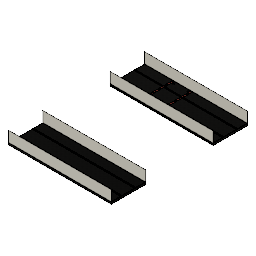
_6-9 (Long Straight 2).344d3e92-f278-4324-a628-1e91485c0ac5 (Autodesk Fusion 360 design; units mm, degrees)
Autodesk Fusion 360 part; units mm, degrees
note: some values were not read from the file. Chosen so that the rebuilt part matches the saved one: which bodies a step acts on.
sketch "Sketch1" plane through (0, 0, 0) normal (0, 0, 1) x (1, 0, 0)
  line L0 (0, 0) -> (0, -812.8)
  line L1 (0, -812.8) -> (0, -2413)
  line L2 (0, -2413) -> (0, -3225.8)
  line L3 (0, 0) -> (1219.2, 0)
  line L4 (1219.2, 0) -> (0, 0)
  line L5 (0, 0) -> (0, -812.8)
  line L6 (0, -812.8) -> (1219.2, -812.8)
  line L7 (1219.2, -812.8) -> (1219.2, 0)
  line L8 (0, -3225.8) -> (1219.2, -3225.8)
  line L9 (1219.2, -3225.8) -> (0, -3225.8)
  line L10 (0, -3225.8) -> (0, -2413)
  line L11 (0, -2413) -> (1219.2, -2413)
  line L12 (1219.2, -2413) -> (1219.2, -3225.8)
  dimension "d1" = 812.8
  dimension "d2" = 1600.2
  dimension "d3" = 812.8
  dimension "d4" = 1219.2
  dimension "d5" = 1219.2
  constraint coincident L0.start L3.start
  constraint vertical L0
  constraint parallel L0 L1
  constraint parallel L1 L2
  constraint perpendicular L0 L3
  constraint horizontal L4
  constraint vertical L5
  constraint horizontal L6
  constraint vertical L7
  constraint perpendicular L2 L8
  constraint horizontal L9
  constraint vertical L10
  constraint horizontal L11
  constraint vertical L12
  measures "d1" distance of L0.start L0.end
  measures "d2" distance of L0.end L1.end
  measures "d3" distance of L1.end L2.end
  measures "d4" distance of L0.start L3.end
  measures "d5" distance of L2.end L8.end
extrude "Extrude1" add sketch "Sketch1" along normal blind 50.8 makes body 1 at (406.4, -270.9333, 0) makes body 2 at (812.8, -2954.8667, 0)
sketch "Sketch2" plane through (0, 0, 50.8) normal (0, 0, 1) x (-1, 0, 0)
  line L0 (-1219.2, 2413) -> (0, 2413)
  line L1 (0, 2413) -> (0, 3225.8)
  line L2 (0, 3225.8) -> (-1219.2, 3225.8)
  line L3 (-1219.2, 3225.8) -> (-1219.2, 2413)
  line L4 (-106.2446, 261.963) -> (-283.0518, 261.963) construction
  line L5 (-283.0518, 261.963) -> (-283.0518, 108.5567) construction
  line L6 (-283.0518, 108.5567) -> (-106.2446, 108.5567) construction
  line L7 (-106.2446, 108.5567) -> (-106.2446, 261.963) construction
  dimension "d8" = 152.4
sketch "Sketch3" plane through (0, 0, 50.8) normal (0, 0, 1) x (-1, 0, 0)
  line L0 (-1219.2, 812.8) -> (-1219.2, 0)
  line L1 (-1219.2, 0) -> (0, 0)
  line L2 (0, 0) -> (0, 812.8)
  line L3 (0, 812.8) -> (-1219.2, 812.8)
  line L4 (-1219.2, 406.4) -> (-1139.825, 406.4)
  line L5 (-1139.825, 406.4) -> (-1111.25, 406.4)
  line L6 (-1111.25, 406.4) -> (-1111.25, 0)
  line L7 (-1111.25, 0) -> (-1139.825, 0)
  line L8 (-1139.825, 0) -> (-1139.825, 406.4)
  line L9 (-1139.825, 406.4) -> (-1111.25, 406.4)
  line L10 (-1111.25, 406.4) -> (-1111.25, 812.8)
  line L11 (-1111.25, 812.8) -> (-1139.825, 812.8)
  line L12 (-1139.825, 812.8) -> (-1139.825, 406.4)
  line L13 (-1219.2, 406.4) -> (-704.85, 406.4)
  line L14 (-704.85, 406.4) -> (-676.275, 406.4)
  line L15 (-676.275, 406.4) -> (-676.275, 0)
  line L16 (-676.275, 0) -> (-704.85, 0)
  line L17 (-704.85, 0) -> (-704.85, 406.4)
  line L18 (-676.275, 406.4) -> (-704.85, 406.4)
  line L19 (-704.85, 406.4) -> (-704.85, 812.8)
  line L20 (-704.85, 812.8) -> (-676.275, 812.8)
  line L21 (-676.275, 812.8) -> (-676.275, 406.4)
  dimension "d9" = 79.375
  dimension "d10" = 28.575
  dimension "d11" = 28.575
  dimension "d12" = 514.35
  dimension "d13" = 28.575
  dimension "d14" = 28.575
  constraint midpoint L0 L4.start
  constraint perpendicular L0 L4
  constraint horizontal L5
  constraint vertical L6
  constraint horizontal L7
  constraint vertical L8
  constraint coincident L1 L6.end
  constraint horizontal L9
  constraint vertical L10
  constraint horizontal L11
  constraint vertical L12
  constraint coincident L3 L10.end
  constraint perpendicular L12 L13
  constraint horizontal L14
  constraint vertical L15
  constraint horizontal L16
  constraint vertical L17
  constraint horizontal L18
  constraint vertical L19
  constraint horizontal L20
  constraint vertical L21
  measures "d9" distance of L4.start L4.end
  measures "d10" distance of L4.end L5.end
  measures "d11" distance of L4.end L5.end
  measures "d12" distance of L4.start L13.end
  measures "d13" distance of L13.end L14.end
  measures "d14" distance of L14.end L13.end
extrude "Extrude2" add sketch "Sketch3" along normal blind 0.0254 contours L3 L5 L9 L10 L11 L12 L13 | L1 L5 L6 L7 L8 L9 L13 | L3 L14 L18 L19 L20 L21 | L1 L14 L15 L16 L17 L18 bodies 1
sketch "Sketch4" plane through (0, 0, 50.8) normal (0, 0, 1) x (-1, 0, 0)
  line L0 (-676.275, 812.8) -> (-676.275, 0)
  line L1 (-676.275, 0) -> (0, 0)
  line L2 (0, 0) -> (0, 812.8)
  line L3 (0, 812.8) -> (-676.275, 812.8)
  line L4 (-1111.25, 812.8) -> (-1111.25, 0)
  line L5 (-1111.25, 0) -> (-704.85, 0)
  line L6 (-704.85, 0) -> (-704.85, 812.8)
  line L7 (-704.85, 812.8) -> (-1111.25, 812.8)
  line L8 (-1139.825, 0) -> (-1139.825, 812.8)
  line L9 (-1139.825, 812.8) -> (-1219.2, 812.8)
  line L10 (-1219.2, 812.8) -> (-1219.2, 0)
  line L11 (-1219.2, 0) -> (-1139.825, 0)
  line L12 (-704.85, 0) -> (-1111.25, 0)
  line L13 (-1111.25, 0) -> (-1111.25, 57.15)
  line L14 (-704.85, 57.15) -> (-704.85, 0)
  line L15 (-704.85, 812.8) -> (-1111.25, 812.8)
  line L16 (-1111.25, 812.8) -> (-1111.25, 755.65)
  line L17 (-704.85, 755.65) -> (-704.85, 812.8)
  circle A0 centre (-742.95, 57.15) radius 16
  circle A1 centre (-1085.85, 57.15) radius 16
  circle A2 centre (-742.95, 755.65) radius 16
  circle A3 centre (-1085.85, 755.65) radius 16
  dimension "d19" = 57.15
  dimension "d20" = 57.15
  dimension "d21" = 32
  dimension "d22" = 32
  dimension "d23" = 32
  dimension "d24" = 32
  constraint horizontal L12
  constraint vertical L13
  constraint vertical L14
  constraint coincident L5.end L6.start
  constraint horizontal L15
  constraint vertical L16
  constraint vertical L17
  constraint coincident L6.end L7.start
  measures "d19" distance of L5.end L14.start
  measures "d20" distance of L6.end L17.start
  measures "d21" diameter of A0
  measures "d22" diameter of A1
  measures "d23" diameter of A2
  measures "d24" diameter of A3
extrude "Extrude3" add sketch "Sketch4" along normal blind 0.0254 contours A0 | A1 | A2 | A3 bodies 1
sketch "Sketch5" plane through (0, 0, 50.8) normal (0, 0, 1) x (-1, 0, 0)
sketch "Sketch6" plane through (0, 0, 50.8) normal (0, 0, 1) x (-1, 0, 0)
  line L0 (-676.275, 812.8) -> (-676.275, 0)
  line L1 (-676.275, 0) -> (0, 0)
  line L2 (0, 0) -> (0, 812.8)
  line L3 (0, 812.8) -> (-676.275, 812.8)
  line L4 (-676.275, 250.825) -> (0, 250.825)
  line L5 (-676.275, 231.775) -> (0, 231.775)
  line L6 (0, 561.975) -> (-676.275, 561.975)
  line L7 (0, 581.025) -> (-676.275, 581.025)
  dimension "d27" = -250.825
  dimension "d28" = -231.775
  dimension "d29" = -250.825
  dimension "d30" = -231.775
extrude "Extrude4" add sketch "Sketch6" along normal blind 0.0279 contours L0 L2 L4 L5 bodies 1
extrude "Extrude5" add sketch "Sketch6" along normal blind 0.0279 contours L0 L2 L6 L7 bodies 1
sketch "Sketch7" plane through (0, 0, 50.8) normal (0, 0, 1) x (-1, 0, 0)
  circle A0 centre (-742.95, 755.65) radius 16
  circle A1 centre (-742.95, 57.15) radius 16
  circle A2 centre (-1085.85, 755.65) radius 16
  circle A3 centre (-1085.85, 57.15) radius 16
  line L0 (-1111.25, 812.8) -> (-1111.25, 0)
  line L1 (-1111.25, 0) -> (-704.85, 0)
  line L2 (-704.85, 0) -> (-704.85, 812.8)
  line L3 (-704.85, 812.8) -> (-1111.25, 812.8)
  line L4 (-1111.25, 250.825) -> (-704.85, 250.825)
  line L5 (-1111.25, 231.775) -> (-704.85, 231.775)
  line L6 (-704.85, 561.975) -> (-1111.25, 561.975)
  line L7 (-704.85, 581.025) -> (-1111.25, 581.025)
  dimension "d35" = -250.825
  dimension "d36" = -231.775
  dimension "d37" = -250.825
  dimension "d38" = -231.775
extrude "Extrude6" add sketch "Sketch7" along normal blind 0.0279 contours L0 L2 L6 L7 | L0 L2 L4 L5 bodies 1
sketch "Sketch8" plane through (0, 0, 50.8) normal (0, 0, 1) x (-1, 0, 0)
  line L0 (-1139.825, 0) -> (-1139.825, 812.8)
  line L1 (-1139.825, 812.8) -> (-1219.2, 812.8)
  line L2 (-1219.2, 812.8) -> (-1219.2, 0)
  line L3 (-1219.2, 0) -> (-1139.825, 0)
  line L4 (-1219.2, 250.825) -> (-1139.825, 250.825)
  line L5 (-1219.2, 231.775) -> (-1139.825, 231.775)
  line L6 (-1139.825, 561.975) -> (-1219.2, 561.975)
  line L7 (-1139.825, 581.025) -> (-1219.2, 581.025)
  dimension "d41" = -250.825
  dimension "d42" = -231.775
  dimension "d43" = -250.825
  dimension "d44" = -231.775
extrude "Extrude7" add sketch "Sketch8" along normal blind 0.0279 contours L0 L2 L6 L7 bodies 1
extrude "Extrude8" add sketch "Sketch8" along normal blind 0.0279 contours L0 L2 L4 L5 bodies 1
sketch "Sketch9" plane through (0, 0, 50.8) normal (0, 0, 1) x (-1, 0, 0)
  line L0 (-1219.2, 2413) -> (0, 2413)
  line L1 (0, 2413) -> (0, 3225.8)
  line L2 (0, 3225.8) -> (-1219.2, 3225.8)
  line L3 (-1219.2, 3225.8) -> (-1219.2, 2413)
  line L4 (-1219.2, 2663.825) -> (0, 2663.825)
  line L5 (-1219.2, 2644.775) -> (0, 2644.775)
  line L6 (0, 2974.975) -> (-1219.2, 2974.975)
  line L7 (0, 2994.025) -> (-1219.2, 2994.025)
  dimension "d49" = -250.825
  dimension "d50" = -231.775
  dimension "d51" = -250.825
  dimension "d52" = -231.775
extrude "Extrude9" add sketch "Sketch9" along normal blind 0.0279 contours L1 L3 L4 L5 | L1 L3 L6 L7 bodies 2
sketch "Sketch10" plane through (0, 0, 0) normal (0, 0, -1) x (1, 0, 0)
  line L0 (0, 2413) -> (1219.2, 2413)
  line L1 (1219.2, 2413) -> (1219.2, 3225.8)
  line L2 (1219.2, 3225.8) -> (0, 3225.8)
  line L3 (0, 3225.8) -> (0, 2413)
sketch "Sketch11" plane through (0, 0, 0) normal (0, 0, -1) x (1, 0, 0)
  line L0 (1219.2, 0) -> (1219.2, 812.8)
  line L1 (1219.2, 812.8) -> (0, 812.8)
  line L2 (0, 812.8) -> (0, 0)
  line L3 (0, 0) -> (1219.2, 0)
  line L4 (1218.946, 812.546) -> (0.254, 812.546)
  line L5 (0.254, 812.546) -> (0.254, 0.254)
  line L6 (0.254, 0.254) -> (1218.946, 0.254)
  line L7 (1218.946, 0.254) -> (1218.946, 812.546)
  dimension "d55" = -0.254
extrude "Extrude10" add sketch "Sketch11" along normal blind 254 separate body makes body 3
sketch "Sketch12" plane through (0, 0, -254) normal (0, 0, -1) x (1, 0, 0)
  line L0 (1218.946, 812.546) -> (1218.946, 0.254)
  line L1 (1218.946, 0.254) -> (0.254, 0.254)
  line L2 (0.254, 0.254) -> (0.254, 812.546)
  line L3 (0.254, 812.546) -> (1218.946, 812.546)
  line L4 (0, 0) -> (1219.2, 0)
  line L5 (1219.2, 0) -> (1219.2, 812.8)
  line L6 (1219.2, 812.8) -> (0, 812.8)
  line L7 (0, 812.8) -> (0, 0)
  line L8 (0.254, 0.254) -> (0, 0.254)
  line L9 (0.254, 812.546) -> (0, 812.546)
  constraint coincident L1.end L2.start
  constraint coincident L7 L8.end
  constraint perpendicular L7 L8
  constraint coincident L2.end L3.start
  constraint perpendicular L2 L9
extrude "Extrude11" cut sketch "Sketch12" against normal blind 254 contours L2 L7 L8 L9 bodies 3
sketch "Sketch13" plane through (0, 0, -254) normal (0, 0, -1) x (1, 0, 0)
  line L0 (0, 812.546) -> (1218.946, 812.546)
  line L1 (1218.946, 812.546) -> (1218.946, 0.254)
  line L2 (1218.946, 0.254) -> (0, 0.254)
  line L3 (0, 0.254) -> (0, 0)
  line L4 (0, 0) -> (1219.2, 0)
  line L5 (1219.2, 0) -> (1219.2, 812.8)
  line L6 (1219.2, 812.8) -> (0, 812.8)
  line L7 (0, 812.8) -> (0, 812.546)
  line L8 (1218.946, 0.254) -> (1219.2, 0.254)
  line L9 (1218.946, 812.546) -> (1219.2, 812.546)
  constraint coincident L1.end L2.start
  constraint coincident L5 L8.end
  constraint perpendicular L5 L8
  constraint coincident L0.end L1.start
  constraint coincident L5 L9.end
  constraint perpendicular L5 L9
extrude "Extrude12" cut sketch "Sketch13" against normal blind 254 contours L1 L5 L8 L9 bodies 3 makes body 4 at (812.8, -0.254, -169.3333)
move_body "Move1" bodies 3 4 to x (1, 0, 0) y (0, 1, 0) z (0, 0, 1) at (0, 0, 304.8)
sketch "Sketch14" plane through (0, 0, 0) normal (0, 0, -1) x (1, 0, 0)
sketch "Sketch15" plane through (0, 0, 0) normal (0, 0, -1) x (1, 0, 0)
sketch "Sketch16" plane through (0, 0, 0) normal (0, 0, -1) x (1, 0, 0)
  line L0 (0, 2413) -> (1219.2, 2413)
  line L1 (1219.2, 2413) -> (1219.2, 3225.8)
  line L2 (1219.2, 3225.8) -> (0, 3225.8)
  line L3 (0, 3225.8) -> (0, 2413)
  line L4 (-0.254, 2412.746) -> (1219.454, 2412.746)
  line L5 (1219.454, 2412.746) -> (1219.454, 3226.054)
  line L6 (1219.454, 3226.054) -> (-0.254, 3226.054)
  line L7 (-0.254, 3226.054) -> (-0.254, 2412.746)
  dimension "d65" = 0.254
sketch "Sketch17" plane through (0, 0, 0) normal (0, 0, -1) x (1, 0, 0)
sketch "Sketch18" plane through (0, 0, 0) normal (0, 0, -1) x (1, 0, 0)
  line L0 (0, 2413) -> (1219.2, 2413)
  line L1 (1219.2, 2413) -> (1219.2, 3225.8)
  line L2 (1219.2, 3225.8) -> (0, 3225.8)
  line L3 (0, 3225.8) -> (0, 2413)
  line L4 (1219.454, 3226.054) -> (-0.254, 3226.054)
  line L5 (-0.254, 3226.054) -> (-0.254, 2412.746)
  line L6 (-0.254, 2412.746) -> (1219.454, 2412.746)
  line L7 (1219.454, 2412.746) -> (1219.454, 3226.054)
  line L8 (1219.2, 3225.8) -> (1219.454, 3225.8)
  line L9 (1219.2, 2413) -> (1219.454, 2413)
  line L10 (0, 2413) -> (-0.254, 2413)
  line L11 (0, 3225.8) -> (-0.254, 3225.8)
  dimension "d66" = 0.254
  constraint coincident L1.end L2.start
  constraint coincident L7 L8.end
  constraint perpendicular L7 L8
  constraint coincident L0.end L1.start
  constraint coincident L7 L9.end
  constraint perpendicular L7 L9
  constraint coincident L0.start L3.end
  constraint coincident L5 L10.end
  constraint perpendicular L5 L10
  constraint coincident L2.end L3.start
  constraint coincident L5 L11.end
  constraint perpendicular L5 L11
sketch "Sketch19" plane through (0, 0, 50.8) normal (0, 0, 1) x (-1, 0, 0)
  line L0 (0, 2644.775) -> (-1219.2, 2644.775)
  line L1 (-1219.2, 2644.775) -> (-1219.2, 2413)
  line L2 (-1219.2, 2413) -> (0, 2413)
  line L3 (0, 2413) -> (0, 2644.775)
  line L4 (-1219.2, 2413.254) -> (0, 2413.254)
  dimension "d69" = -0.254
extrude "Extrude14" add sketch "Sketch19" along normal blind 254 separate body contours L1 L2 L3 L4 makes body 5
sketch "Sketch20" plane through (0, 0, 50.8) normal (0, 0, 1) x (-1, 0, 0)
  line L0 (-1219.2, 2994.025) -> (0, 2994.025)
  line L1 (0, 2994.025) -> (0, 3225.8)
  line L2 (0, 3225.8) -> (-1219.2, 3225.8)
  line L3 (-1219.2, 3225.8) -> (-1219.2, 2994.025)
  line L4 (0, 3225.546) -> (-1219.2, 3225.546)
  dimension "d72" = -0.254
extrude "Extrude15" add sketch "Sketch20" along normal blind 254 separate body contours L1 L2 L3 L4 makes body 6
copy_body "CopyPasteBodies1" bodies 2 makes body 7
move_body "Move4" bodies 7 to x (1, 0, 0) y (0, 1, 0) z (0, 0, 1) at (1524, 0, 0)
move_body "Align1" bodies 7 to x (1, 0, 0) y (0, 1, 0) z (0, 0, 1) at (-304.8, 0, 0)
copy_body "CopyPasteBodies2" bodies 7 makes body 8
move_body "Move5" bodies 8 to x (1, 0, 0) y (0, 1, 0) z (0, 0, 1) at (0, 2413, 0)
combine "Combine1" operation add target body 1 tool bodies 8
combine "Combine2" operation add target body 2 tool bodies 7
copy_body "CopyPasteBodies3" bodies 6 makes body 9
move_body "Move6" bodies 9 to x (1, 0, 0) y (0, 1, 0) z (0, 0, 1) at (1219.2, 0, 0)
combine "Combine3" operation add target body 6 tool bodies 9
copy_body "CopyPasteBodies4" bodies 5 makes body 10
move_body "Move7" bodies 10 to x (1, 0, 0) y (0, 1, 0) z (0, 0, 1) at (1219.2, 0, 0)
combine "Combine4" operation add target body 5 tool bodies 10
copy_body "CopyPasteBodies5" bodies 3 makes body 11
move_body "Move8" bodies 11 to x (1, 0, 0) y (0, 1, 0) z (0, 0, 1) at (1219.2, 0, 0)
combine "Combine5" operation add target body 3 tool bodies 11
copy_body "CopyPasteBodies6" bodies 4 makes body 12
move_body "Move9" bodies 12 to x (1, 0, 0) y (0, 1, 0) z (0, 0, 1) at (1219.2, 0, 0)
combine "Combine6" operation add target body 4 tool bodies 12
equation "d4 = ( 24 * 2 ) * 1 in"
equation "d5 = ( 24 * 2 ) * 1 in"
